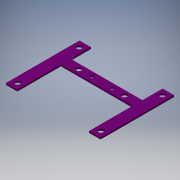
# Autodesk Inventor part: Side
Saved by Autodesk Inventor 2016 (Build 200138000, 138)
## iProperties
Created: 2015-03-28
Part Number: Side
Material: PC/ABS Plastic
Document SubType Name: Modeling
Designer: Erin
Density: 0.357273 g/cm^3
Appearance: Smooth - Purple
Mass: 3.07089 g
Surface Area: 62.8323 cm^2
Volume: 5.58344 cm^3
Author: Erin
Autodesk Inventor part; units mm, degrees
ref_plane "YZ Plane" through (0, 0, 0) normal (1, 0, 0) x (0, 1, 0)
ref_plane "XZ Plane" through (0, 0, 0) normal (0, 1, 0) x (-1, 0, 0)
ref_plane "XY Plane" through (0, 0, 0) normal (0, 0, 1) x (1, 0, 0)
sketch "Sketch1" plane through (0, 0, 0) normal (0, 0, 1) x (1, 0, 0)
  line L0 (-41.5, 50) -> (41.5, 50)
  line L1 (41.5, 50) -> (41.5, -50)
  line L2 (41.5, -50) -> (-41.5, -50)
  line L3 (-41.5, -50) -> (-41.5, 50)
  line L4 (31.5, 40) -> (-31.5, 40)
  line L5 (-31.5, 40) -> (-31.5, -40)
  line L6 (-31.5, -40) -> (31.5, -40)
  line L7 (31.5, -40) -> (31.5, 40)
  line L8 (-41.5, -45) -> (41.5, -45) construction
  line L9 (0, 71.7466) -> (0, -78.0681) construction
  line L10 (-60.2597, 0) -> (74.2823, 0) construction
  line L11 (-36.5, 50) -> (-36.5, -50) construction
  circle A0 centre (-36.5, -27) radius 2.25
  line L12 (-41.5, 45) -> (41.5, 45) construction
  circle A1 centre (-36.5, 45) radius 2.25
  circle A2 centre (-36.5, -45) radius 2.25
  circle A3 centre (-36.5, 27) radius 2.25
  circle A4 centre (-25, -45) radius 2.25
  circle A5 centre (25, -45) radius 2.25
  line L13 (30, 50) -> (30, -50) construction
  line L14 (-30, 50) -> (-30, -50) construction
  line L15 (-31, -38) -> (31, -38)
  line L16 (31, -38) -> (31, -52)
  line L17 (31, -52) -> (-31, -52)
  line L18 (-31, -52) -> (-31, -38)
  line L19 (-31.5, -40) -> (-16.5, -40)
  line L20 (-16.5, -40) -> (-16.5, -20)
  line L21 (-16.5, -20) -> (-31.5, -20)
  line L22 (-31.5, -20) -> (-31.5, -40)
  line L23 (-26.5, -26) -> (-21.5, -26) construction
  line L24 (-26.5, -27.5) -> (-21.5, -27.5)
  line L25 (-21.5, -24.5) -> (-26.5, -24.5)
  arc A6 (-26.5, -24.5) -> (-26.5, -27.5) centre (-26.5, -26) ccw
  arc A7 (-21.5, -27.5) -> (-21.5, -24.5) centre (-21.5, -26) ccw
  line L26 (-26.5, -34) -> (-21.5, -34) construction
  line L27 (-26.5, -35.5) -> (-21.5, -35.5)
  line L28 (-21.5, -32.5) -> (-26.5, -32.5)
  arc A8 (-26.5, -32.5) -> (-26.5, -35.5) centre (-26.5, -34) ccw
  arc A9 (-21.5, -35.5) -> (-21.5, -32.5) centre (-21.5, -34) ccw
  point P0 (0, 0)
  point P1 (0, 50)
  point P2 (41.5, 0)
  point P3 (0, 45)
  point P4 (-24, -26)
  point P5 (-24, -20)
  point P6 (-16.5, -30)
  point P7 (-24, -34)
  dimension "d0" = 83
  dimension "d1" = 100
  dimension "d5" = 5
  dimension "d6" = 5
  dimension "d9" = 5
  dimension "d12" = 4.5
  dimension "d17" = 5
  dimension "d41" = 4.5
  dimension "d42" = 4.5
  dimension "d87" = 4.5
  dimension "d89" = 4.5
  dimension "d90" = 4.5
  dimension "d91" = 30
  dimension "d92" = 30
  dimension "d93" = 5
  dimension "d94" = 5
  dimension "d97" = 1
  dimension "d98" = 2
  dimension "d99" = 2
  dimension "d100" = 1
  dimension "d103" = 15
  dimension "d104" = 20
  dimension "d105" = 5
  dimension "d106" = 3
  dimension "d109" = 5
  dimension "d110" = 3
  dimension "d112" = 6
  dimension "d113" = 6
  dimension "d141" = 27
  dimension "d142" = 27
  constraints: 62 end point, 18 point on line, 11 perpendicular, 10 centre point, 10 parallel, 8 point on circle, 8 tangent, 7 midpoint, 4 horizontal, 3 vertical alignment, 1 horizontal alignment, 1 vertical, 3 other
  measures "d0" distance of L1.end L2.end
  measures "d1" distance of L0.end L1.end
  measures "d5" distance between parallel lines of L8 L2
  measures "d6" distance between parallel lines of L6 L8
  measures "d9" distance between parallel lines of L11 L3
  measures "d12" diameter of A0
  measures "d17" distance between parallel lines of L12 L0
  measures "d41" diameter of A1
  measures "d42" diameter of A2
  measures "d87" diameter of A3
  measures "d89" diameter of A4
  measures "d90" diameter of A5
  measures "d91" distance between parallel lines of L13 L9
  measures "d92" distance between parallel lines of L14 L9
  measures "d93" distance from line of A4.centre L14
  measures "d94" distance from line of A5.centre L13
  measures "d97" distance between parallel lines of L14 L18
  measures "d98" distance between parallel lines of L2 L17
  measures "d99" distance between parallel lines of L6 L15
  measures "d100" distance between parallel lines of L13 L16
  measures "d103" distance of L21.end L20.end
  measures "d104" distance of L20.end L19.end
  measures "d105" distance of L25.start L25.end
  measures "d106" distance between parallel lines of L24 L25
  measures "d109" distance of L28.start L28.end
  measures "d110" distance between parallel lines of L27 L28
  measures "d112" distance between parallel lines of L26 L19
  measures "d113" distance between parallel lines of L21 L23
  measures "d141" distance from line of A3.centre L10
  measures "d142" distance from line of A0.centre L10
sketch "Sketch4" plane through (0, 0, 0) normal (0, 0, 1) x (1, 0, 0)
  circle A0 centre (-36.5, 27) radius 2.25 projected
  circle A1 centre (-36.5, -27) radius 2.25 projected
  line L0 (-31.5, 40) -> (-31.5, -40) projected
  line L1 (-41.5, -50) -> (-41.5, 50) projected
  line L2 (-41.5, -32.25) -> (-31.5, -32.25)
  line L3 (-31.5, -32.25) -> (-31.5, 32.25)
  line L4 (-31.5, 32.25) -> (-41.5, 32.25)
  line L5 (-41.5, 32.25) -> (-41.5, -32.25)
  line L6 (31.5, -40) -> (31.5, 40) projected
  line L7 (41.5, 50) -> (41.5, -50) projected
  line L8 (31.5, -18) -> (31.5, 0)
  line L9 (-31.5, 0) -> (-31.5, -18)
  line L10 (-16.5, -20) -> (-31.5, -20) projected
  line L11 (-31.5, -40) -> (31.5, -40) projected
  line L12 (-16.5, -40) -> (-16.5, -20) projected
  line L13 (-31.5, 14.5) -> (0, 14.5)
  line L14 (0, 14.5) -> (0, 6)
  line L15 (0, 6) -> (-31.5, 6)
  line L16 (-31.5, 6) -> (-31.5, 14.5)
  circle A2 centre (-9, 10.25) radius 1.5
  line L17 (0, 10.25) -> (-31.5, 10.25) construction
  circle A3 centre (-20, 10.25) radius 2.25
  line L18 (0, 28.3973) -> (0, -18) construction
  point P0 (0, 0)
  dimension "d116" = 3
  dimension "d117" = 3
  dimension "d151" = 8.5
  dimension "d152" = 3
  dimension "d153" = 9
  dimension "d154" = 22
  dimension "d155" = 4.5
  dimension "d156" = 20
  constraints: 24 end point, 5 parallel, 5 point on line, 3 midpoint, 2 centre point, 2 horizontal, 2 perpendicular, 2 vertical, 1 horizontal alignment
  measures "d116" distance edge to line of A0 L4
  measures "d117" distance edge to line of A1 L2
  measures "d151" distance of L13.end L14.end
  measures "d152" diameter of A2
  measures "d153" distance from line of A2.centre L14
  measures "d154" distance between parallel lines of L17 L4
  measures "d155" diameter of A3
  measures "d156" distance from line of L18 A3.centre
extrude "Extrusion11" add sketch "Sketch4" along normal blind 1.5 contours L0 L2 L1 L4 | L13 L14 L15 L0
mirror "Mirror10" about plane through (0, 0, 0) normal (1, 0, 0) of "Extrusion11"
equation "\"d12\" = screw"
equation "\"d41\" = screw"
equation "\"d42\" = screw"
equation "\"d87\" = screw"
equation "\"d89\" = screw"
equation "\"d90\" = screw"
equation "\"screw\" = 4.5"
body "Solid2"
